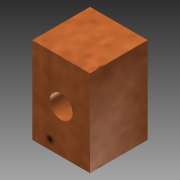
# Autodesk Inventor part: panGearSpacerBlocks
Saved by Autodesk Inventor 2013 (Build 170138000, 138)
## iProperties
Created: 2014-06-30
Part Number: panGearSpacerBlocks
Material: Wood (Cherry)
Document SubType Name: Modeling
Designer: Nano
Mass: 1.41014 g
Surface Area: 14.5125 cm^2
Volume: 2.82029 cm^3
Density: 0.5 g/cm^3
Author: Nano
Autodesk Inventor part; units mm, degrees
ref_plane "YZ Plane" through (0, 0, 0) normal (1, 0, 0) x (0, 1, 0)
ref_plane "XZ Plane" through (0, 0, 0) normal (0, 1, 0) x (-1, 0, 0)
ref_plane "XY Plane" through (0, 0, 0) normal (0, 0, 1) x (1, 0, 0)
ref_plane "Work Plane1" through (0, 0, 0) normal (0, 0, 1) x (1, 0, 0)
sketch "Sketch1" plane through (0, 0, 0) normal (0, 0, 1) x (1, 0, 0)
  circle A0 centre (38.1, -88.9) radius 2.5146 projected
  line L0 (44.45, -98.425) -> (31.75, -98.425)
  line L1 (31.75, -98.425) -> (31.75, -79.375)
  line L2 (31.75, -79.375) -> (44.45, -79.375)
  line L3 (44.45, -79.375) -> (44.45, -98.425)
  point P0 (0, 0)
  dimension "d0" = 19.05
  dimension "d2" = 12.7
  dimension "d3" = 9.525
  dimension "d4" = 9.525
  dimension "d5" = 6.35
  dimension "d6" = 6.35
  constraints: 8 end point, 2 parallel, 1 horizontal, 1 perpendicular
  measures "d0" distance of L2.end L0.start
  measures "d2" distance of L0.start L0.end
  measures "d3" distance from line of L2 A0.centre
  measures "d4" distance from line of L0 A0.centre
  measures "d5" distance from line of L3 A0.centre
  measures "d6" distance from line of L1 A0.centre
extrude "Extrusion1" add sketch "Sketch1" along normal blind 13.716
equation "\"d3\" = d4"
equation "\"d5\" = d6"
body "Solid1"
